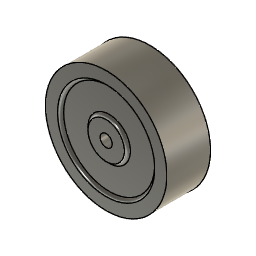
Upper Rolling Wheel (Autodesk Fusion 360 design; units mm, degrees)
Autodesk Fusion 360 part; units mm, degrees
sketch "Sketch1" plane through (0, 0, 0) normal (0, 1, 0) x (1, 0, 0)
  circle A0 centre (0, 0) radius 63.5
  circle A1 centre (0, 0) radius 6.35
  constraint coincident A0.centre A1.centre
  constraint concentric A0 A1
extrude "Extrude1" add sketch "Sketch1" along normal blind 45.72 makes body 1
sketch "Sketch2" plane through (0, 0, 0) normal (0, -1, 0) x (1, 0, 0)
  circle A0 centre (0, 0) radius 6.35
  circle A1 centre (0, 0) radius 63.5
  circle A2 centre (0, 0) radius 50.8
  circle A3 centre (0, 0) radius 19.05
  dimension "d5" = 101.6
  dimension "d6" = 38.1
  constraint concentric A0 A2
  constraint concentric A2 A3
  measures "d5" diameter of A2
  measures "d6" diameter of A3
extrude "Extrude2" cut sketch "Sketch2" against normal blind 3.175 contours A2 bodies 1
sketch "Sketch3" plane through (0, 45.72, 0) normal (0, 1, 0) x (-1, 0, 0)
  circle A0 centre (0, 0) radius 6.35
  circle A1 centre (0, 0) radius 63.5
  circle A2 centre (0, 0) radius 50.8
  circle A3 centre (0, 0) radius 19.05
  dimension "d9" = 101.6
  dimension "d10" = 38.1
  constraint concentric A0 A2
  constraint concentric A2 A3
  measures "d9" diameter of A2
  measures "d10" diameter of A3
extrude "Extrude3" cut sketch "Sketch3" against normal blind 3.175 contours A2 bodies 1
fillet "Fillet1" radius 3.175 2 edges at (17.7608, 42.545, -6.8888) (47.3622, 42.545, 18.3701) on bodies 1
fillet "Fillet2" radius 3.175 2 edges at (-17.7608, 3.175, -6.8888) (-47.3622, 3.175, 18.3701) on bodies 1
copy_body "Body->Comp1" bodies 1 removing the originals makes body 2 in component "Rolling Wheel"
component "Rolling Wheel" placed x (1, 0, 0) y (0, 1, 0) z (0, 0, 1) at (0, 0, 0)
equation "d7 = ( -1 / 4 / 2 ) * 1 in"
named bodies: "Rolling Wheel"
